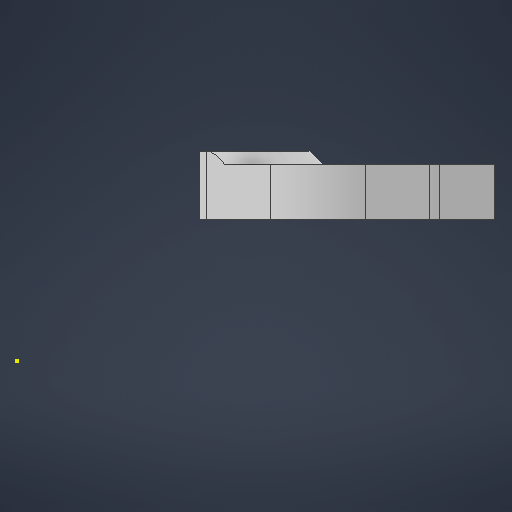
# Autodesk Inventor part: guideline_mir
Saved by Autodesk Inventor 2026 (Build 300175000, 175)
## iProperties
Created: 2025-11-28
Part Number: guideline_mir
Material: 一般
Document SubType Name: Modeling
Designer: numai
Density: 1 g/cm^3
Appearance: 既定
Author: numai
Autodesk Inventor part; units mm, degrees
ref_plane "YZ Plane" through (0, 0, 0) normal (1, 0, 0) x (0, 1, 0)
ref_plane "XZ Plane" through (0, 0, 0) normal (0, 1, 0) x (-1, 0, 0)
ref_plane "XY Plane" through (0, 0, 0) normal (0, 0, 1) x (1, 0, 0)
sketch "スケッチ1" plane through (0, 0, 0) normal (0, 0, 1) x (1, 0, 0)
  circle A0 centre (0, 0) radius 17.3 construction
  line L0 (0, 0) -> (0, 20.4) construction
  circle A1 centre (0, -17.3) radius 3 construction
  circle A2 centre (0, 0) radius 14.3 construction
  circle A3 centre (0, 0) radius 20.3 construction
  circle A4 centre (0, 17.3) radius 3 construction
  circle A5 centre (-8.65, 14.9822) radius 3 construction
  line L1 (-8.65, 14.9822) -> (0, 17.3) construction
  line L2 (-8.65, 14.9822) -> (0, 0) construction
  line L3 (-8.65, 14.9822) -> (8.65, 14.9822) construction
  line L4 (0, 0) -> (8.65, 14.9822) construction
  line L5 (0, 17.3) -> (8.65, 14.9822) construction
  circle A6 centre (8.65, 14.9822) radius 3 construction
  arc A7 (-33.421, 8.3449) -> (33.421, 8.3449) centre (0, 17.3) ccw construction
  line L6 (-8.65, 14.9822) -> (-33.421, 8.3449) construction
  line L7 (8.65, 14.9822) -> (33.421, 8.3449) construction
  arc A8 (-8.65, 14.9822) -> (8.65, 14.9822) centre (0, 17.3) ccw construction
  circle A9 centre (0, 8.3449) radius 3 construction
  line L8 (3, 8.3449) -> (3, -17.3) construction
  line L9 (-3, 8.3449) -> (-3, -17.3) construction
  line L10 (0, -20.3) -> (0, -26) construction
  circle A10 centre (0, 17.3) radius 15.3358 construction
  circle A11 centre (0, 17.3) radius 7 construction
  line L11 (-4.9497, 22.2497) -> (4.9497, 22.2497) construction
  line L12 (4.9497, 22.2497) -> (4.9497, 12.3503) construction
  line L13 (4.9497, 12.3503) -> (-4.9497, 12.3503) construction
  line L14 (-4.9497, 12.3503) -> (-4.9497, 22.2497) construction
  circle A12 centre (0, 17.3) radius 1.5
  line L15 (0, 8.3449) -> (0, -17.7) construction
  arc A13 (3, 8.3449) -> (-3, 8.3449) centre (0, 8.3449) ccw
  line L16 (0, 17.3) -> (0, -17.7) construction
  line L17 (-7.5, 17.3) -> (-7.5, -17.7) construction
  line L18 (7.5, -17.7) -> (7.5, 17.3) construction
  arc A14 (7.5, 17.3) -> (-7.5, 17.3) centre (0, 17.3) ccw construction
  arc A15 (-7.5, -17.7) -> (7.5, -17.7) centre (0, -17.7) ccw
  circle A16 centre (4.9497, 22.2497) radius 1.25
  circle A17 centre (-4.9497, 22.2497) radius 1.25
  circle A18 centre (-4.9497, 12.3503) radius 1.25
  circle A19 centre (4.9497, 12.3503) radius 1.25
  circle A20 centre (0, 17.3) radius 20 construction
  circle A21 centre (0, -17.7) radius 35 construction
  arc A22 (15.3498, 21.9312) -> (-15.3498, 21.9312) centre (0, -17.7) ccw construction
  line L19 (17, 34.8) -> (-17, 34.8)
  line L20 (17, 34.8) -> (17, 26.8) construction
  line L21 (-17, 34.8) -> (-17, 26.8) construction
  line L22 (17, 26.8) -> (-17, 26.8) construction
  line L23 (17, 30.8) -> (-17, 30.8) construction
  line L24 (-13, 26.8) -> (-13, 34.8) construction
  line L25 (13, 26.8) -> (13, 34.8) construction
  circle A23 centre (13, 30.8) radius 1.25
  circle A24 centre (0, 30.8) radius 1.25
  circle A25 centre (-13, 30.8) radius 1.25
  arc A26 (-3, -17.7) -> (3, -17.7) centre (0, -17.7) ccw
  line L26 (-3, -17.7) -> (-3, 8.3449)
  line L27 (3, 8.3449) -> (3, -17.7)
  circle A27 centre (-13, 30.8) radius 4 construction
  circle A28 centre (13, 30.8) radius 4 construction
  line L28 (-16.9264, 30.0362) -> (-7.362, -19.1321)
  line L29 (7.362, -19.1321) -> (16.9264, 30.0362)
  line L30 (-17, 34.8) -> (-17, 30.8)
  arc A29 (-17, 30.8) -> (-16.9264, 30.0362) centre (-13, 30.8) ccw
  arc A30 (16.9264, 30.0362) -> (17, 30.8) centre (13, 30.8) ccw
  line L31 (17, 30.8) -> (17, 34.8)
  point P0 (-5.7522, 15.7587)
  point P1 (-2.8978, 16.5235)
  point P2 (0, -4.6776)
  point P3 (0, -0.2)
  point P4 (0, 24.8)
  point P5 (0, 10.2)
  point P6 (0, -17.3)
  point P7 (0, 34.8)
  dimension "d0" = 34.6
  dimension "d2" = 6
  dimension "d4" = 2.9551
  dimension "d5" = 150
  dimension "d8" = 14
  dimension "d11" = 3
  dimension "d14" = 2.5
  dimension "d15" = 17.3
  dimension "d16" = 40
  dimension "d17" = 10.2
  dimension "d18" = 17.5
  dimension "d19" = 8
  dimension "d20" = 4
  dimension "d21" = 4
  dimension "d22" = 4
  dimension "d23" = 2.5
  dimension "d40" = 0.4
  dimension "d41" = 4.5
  dimension "d44" = 26
  constraints: 70 end point, 39 point on circle, 27 centre point, 20 coincident, 17 tangent, 12 point on line, 9 midpoint, 7 equal radius, 7 vertical, 6 perpendicular, 5 horizontal, 4 vertical alignment, 3 parallel, 1 collinear, 1 concentric, 14 other
  measures "d0" diameter of A0
  measures "d2" diameter of A1
  measures "d4" distance of point (-5.752, 15.759) point (-2.898, 16.524)
  measures "d5" angle of L5 L1
  measures "d8" diameter of A11
  measures "d11" diameter of A12
  measures "d14" diameter of A16
  measures "d15" distance of L1.end point (0, 0)
  measures "d16" diameter of A20
  measures "d17" distance of point (0, 10.2) point (0, 0)
  measures "d18" distance from line of L19 L1.end
  measures "d19" distance between parallel lines of L19 L22
  measures "d20" distance between parallel lines of L19 L23
  measures "d21" distance between parallel lines of L21 L24
  measures "d22" distance between parallel lines of L25 L20
  measures "d23" diameter of A23
  measures "d40" distance of point (0, -17.3) A26.centre
  measures "d41" radial gap between concentric circles of A26 A15
  measures "d44" distance of A28.centre A25.centre
extrude "押し出し1" add sketch "スケッチ1" along normal blind 4 contours L28 A29 L30 L19 L31 A30 L29 A15 | A16 | A17 | A18 | A19
sketch "スケッチ2" plane through (0, 0, 4) normal (0, 0, 1) x (1, 0, 0)
  arc A0 (-7.362, -19.1321) -> (7.362, -19.1321) centre (0, -17.7) ccw projected
  line L0 (17, 34.8) -> (-17, 34.8) projected
  arc A1 (3, 8.3449) -> (-3, 8.3449) centre (0, 8.3449) ccw projected
  circle A2 centre (0, 17.3) radius 1.5 projected
  circle A3 centre (-13, 30.8) radius 1.25 projected
  circle A4 centre (0, 30.8) radius 1.25 projected
  circle A5 centre (13, 30.8) radius 1.25 projected
  circle A6 centre (0, 17.3) radius 10
  circle A7 centre (0, 17.3) radius 4
  line L1 (0, 17.3) -> (0, 34.8) construction
  line L2 (19.8551, 26.8) -> (-19.8551, 26.8)
  line L3 (-16.9264, 30.0362) -> (-7.362, -19.1321) projected
  line L4 (7.362, -19.1321) -> (16.9264, 30.0362) projected
  arc A8 (16.9264, 30.0362) -> (17, 30.8) centre (13, 30.8) ccw projected
  line L5 (17, 30.8) -> (17, 34.8) projected
  line L6 (-17, 34.8) -> (-17, 30.8) projected
  arc A9 (-17, 30.8) -> (-16.9264, 30.0362) centre (-13, 30.8) ccw projected
  line L7 (-3, -17.7) -> (-3, 8.3449) projected
  line L8 (3, 8.3449) -> (3, -17.7) projected
  arc A10 (-3, -17.7) -> (3, -17.7) centre (0, -17.7) ccw projected
  circle A11 centre (0, 17.3) radius 17 construction
  circle A12 centre (16.4207, 12.9) radius 7.5 construction
  line L9 (1.8512, 13.7542) -> (12.9497, 19.5485)
  line L10 (-1.8512, 13.7542) -> (-12.9497, 19.5485)
  arc A13 (15.0265, 20.2693) -> (12.9497, 19.5485) centre (16.4207, 12.9) ccw
  arc A14 (-12.9497, 19.5485) -> (-15.0265, 20.2693) centre (-16.4207, 12.9) ccw
  point P0 (0, 0)
  point P1 (6.8841, 24.5532)
  point P2 (16.2935, 29.35)
  point P3 (-1.8512, 13.7542)
  point P4 (-15.0265, 20.2693)
  point P5 (16.2969, 26.8)
  point P6 (-16.2969, 26.8)
  dimension "d24" = 20
  dimension "d25" = 8
  dimension "d42" = 34
  dimension "d29" = 8
  dimension "d43" = 15
  dimension "d46" = 13.9
  constraints: 8 end point, 6 point on circle, 4 coincident, 4 symmetric about line, 3 centre point, 1 midpoint, 1 parallel, 1 point on line, 1 tangent, 11 other
  measures "d29" distance between parallel lines of L2 L0
  measures "d43" diameter of A12
  measures "d46" distance from line of L2 A12.centre
extrude "押し出し2" add sketch "スケッチ2" along normal blind 11.3 contours L3 L2 A6 L10 A14 | A13 L9 A6 L2 L4 | L2 A6 L9 A7 L10 | A7
sketch "スケッチ3" plane through (0, 0, 15.3) normal (0, 0, 1) x (1, 0, 0)
  arc A0 (-1.8512, 13.7542) -> (1.8512, 13.7542) centre (0, 17.3) ccw projected
  circle A1 centre (0, 17.3) radius 1.5 projected
  circle A2 centre (0, 17.3) radius 4
  line L0 (1.8512, 13.7542) -> (12.9497, 19.5485) projected
  arc A3 (15.0265, 20.2693) -> (12.9497, 19.5485) centre (16.4207, 12.9) ccw projected
  line L1 (15.0265, 20.2693) -> (16.2969, 26.8) projected
  line L2 (16.2969, 26.8) -> (-16.2969, 26.8) projected
  line L3 (-16.2969, 26.8) -> (-15.0265, 20.2693) projected
  arc A4 (-12.9497, 19.5485) -> (-15.0265, 20.2693) centre (-16.4207, 12.9) ccw projected
  line L4 (-12.9497, 19.5485) -> (-1.8512, 13.7542) projected
  point P0 (0, 0)
  point P1 (-1.8512, 13.7542)
  point P2 (1.8512, 13.7542)
  constraints: 1 centre point, 1 coincident, 1 concentric
extrude "押し出し3" cut sketch "スケッチ3" against normal blind 1 contours L4 A4 L3 L2 L1 A3 L0 A2
sketch "スケッチ4" plane through (0, 0, 4) normal (0, 0, 1) x (1, 0, 0)
  line L0 (17, 34.8) -> (-17, 34.8) projected
  circle A0 centre (-13, 30.8) radius 1.25 projected
  circle A1 centre (0, 30.8) radius 1.25 projected
  circle A2 centre (13, 30.8) radius 1.25 projected
  line L1 (-16.9264, 30.0362) -> (-16.2969, 26.8) projected
  arc A3 (-7.362, -19.1321) -> (7.362, -19.1321) centre (0, -17.7) ccw projected
  line L2 (7.362, -19.1321) -> (15.0265, 20.2693) projected
  arc A4 (16.9264, 30.0362) -> (17, 30.8) centre (13, 30.8) ccw projected
  line L3 (17, 30.8) -> (17, 34.8) projected
  line L4 (-17, 34.8) -> (-17, 30.8) projected
  arc A5 (-17, 30.8) -> (-16.9264, 30.0362) centre (-13, 30.8) ccw projected
  line L5 (-16.9264, 30.0362) -> (-7.362, -19.1321) projected
  line L6 (-16.7929, 29.35) -> (16.7929, 29.35)
  line L7 (-16.2969, 26.8) -> (16.2969, 26.8) projected
  line L8 (16.2969, 26.8) -> (16.9264, 30.0362) projected
  arc A6 (15.0265, 20.2693) -> (12.9497, 19.5485) centre (16.4207, 12.9) ccw projected
  line L9 (12.9497, 19.5485) -> (1.8512, 13.7542) projected
  arc A7 (-1.8512, 13.7542) -> (1.8512, 13.7542) centre (0, 17.3) ccw projected
  line L10 (-1.8512, 13.7542) -> (-12.9497, 19.5485) projected
  arc A8 (-12.9497, 19.5485) -> (-15.0265, 20.2693) centre (-16.4207, 12.9) ccw projected
  line L11 (-15.0265, 20.2693) -> (-7.362, -19.1321) projected
  point P0 (0, 0)
  point P1 (-16.2935, 29.35)
  point P2 (16.7929, 29.35)
  point P3 (13.4899, 29.35)
  point P4 (12.5101, 29.35)
  point P5 (0.4899, 29.35)
  point P6 (-0.4899, 29.35)
  point P7 (-12.5101, 29.35)
  point P8 (-13.4899, 29.35)
  constraints: 3 point on line, 2 end point, 1 horizontal
extrude "押し出し4" add sketch "スケッチ4" along normal blind 50.3 contours L3 A4 L8 L6 L1 A5 L4 L0 | L8 L7 L1 L6
sketch "スケッチ5" plane through (0, 0, 0) normal (0, 0, -1) x (-1, 0, 0)
  point P0 (0, 0)
chamfer "面取り1" distance 1 angle 45 1 edges at (0, 21.3, 14.3)
sketch "スケッチ7" plane through (0, 0, 0) normal (0, 0, -1) x (-1, 0, 0)
  line L0 (-28.0546, -51.381) -> (31.0808, -51.381)
  line L1 (31.0808, -51.381) -> (31.0808, 46.7157)
  line L2 (31.0808, 46.7157) -> (-28.0546, 46.7157)
  line L3 (-28.0546, 46.7157) -> (-28.0546, -51.381)
  point P0 (0, 0)
  constraints: 8 end point, 2 parallel, 1 horizontal, 1 perpendicular
extrude "押し出し6" cut sketch "スケッチ7" against normal blind 10.3
sketch "スケッチ8" plane through (0, 0, 54.3) normal (0, 0, 1) x (1, 0, 0)
  line L0 (-16.2969, 26.8) -> (16.2969, 26.8) projected
  line L1 (16.2969, 26.8) -> (16.9264, 30.0362) projected
  arc A0 (16.9264, 30.0362) -> (17, 30.8) centre (13, 30.8) ccw projected
  line L2 (17, 30.8) -> (17, 34.8) projected
  line L3 (17, 34.8) -> (-17, 34.8) projected
  line L4 (-17, 34.8) -> (-17, 30.8) projected
  arc A1 (-17, 30.8) -> (-16.9264, 30.0362) centre (-13, 30.8) ccw projected
  line L5 (-16.9264, 30.0362) -> (-16.2969, 26.8) projected
extrude "押し出し7" cut sketch "スケッチ8" against normal up to surface (40 mm away)
sketch "スケッチ9" plane through (0, 0, 14.3) normal (0, 0, 1) x (1, 0, 0)
  circle A0 centre (-13, 30.8) radius 1.25 projected
  circle A1 centre (0, 30.8) radius 1.25 projected
  circle A2 centre (13, 30.8) radius 1.25 projected
  circle A3 centre (-13, 30.8) radius 1.65
  circle A4 centre (0, 30.8) radius 1.65
  circle A5 centre (13, 30.8) radius 1.65
  point P0 (0, 0)
  dimension "d57" = 3.3
  constraints: 3 centre point, 3 coincident, 2 equal radius
  measures "d57" diameter of A3
extrude "押し出し8" cut sketch "スケッチ9" against normal through all contours A0 | A1 | A2 | A3 | A4 | A5
fillet "フィレット3" radius 10 2 edges at (-15.0265, 20.2693, 12.3) (15.0265, 20.2693, 12.3)
sketch "スケッチ12" plane through (0, 0, 15.3) normal (0, 0, 1) x (1, 0, 0)
  arc A0 (-1.8512, 13.7542) -> (1.8512, 13.7542) centre (0, 17.3) ccw projected
  arc A1 (1.8512, 13.7542) -> (-1.8512, 13.7542) centre (0, 17.3) ccw projected
  circle A2 centre (0, 17.3) radius 1.5 projected
  point P0 (0, 0)
equation "\"d20\" = 0.5 * d19"
equation "\"d21\" = d20"
equation "\"d22\" = d21"
